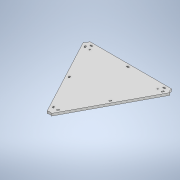
# Autodesk Inventor part: bcc_face
Saved by Autodesk Inventor 2020 (Build 240168000, 168)
## iProperties
Created: 2019-09-26
Part Number: bcc_face
Material: Generic
Document SubType Name: Modeling
Designer: fabrizio
Density: 1 g/cm^3
Appearance: Default
Author: fabrizio
Autodesk Inventor part; units mm, degrees
ref_plane "YZ Plane" through (0, 0, 0) normal (1, 0, 0) x (0, 1, 0)
ref_plane "XZ Plane" through (0, 0, 0) normal (0, 1, 0) x (-1, 0, 0)
ref_plane "XY Plane" through (0, 0, 0) normal (0, 0, 1) x (1, 0, 0)
sketch "Sketch1" plane through (0, 0, 0) normal (0, 1, 0) x (-1, 0, 0)
  arc A0 (8, 0) -> (3.7667, 7.0578) centre (0, 0) ccw
  arc A1 (154.3333, 7.0578) -> (150.1, 0) centre (158.1, 0) ccw
  arc A2 (75.2833, 141.0622) -> (82.8167, 141.0622) centre (79.05, 148.12) ccw
  circle A3 centre (20.0978, 12.0549) radius 1
  circle A4 centre (138.0022, 12.0549) radius 1
  line L0 (3.7667, 7.0578) -> (75.2833, 141.0622)
  line L1 (82.8167, 141.0622) -> (154.3333, 7.0578)
  line L2 (150.1, 0) -> (8, 0)
  line L3 (14.06, 4) -> (17.56, 4)
  line L4 (17.56, 4) -> (17.56, 6)
  line L5 (17.56, 6) -> (14.06, 6)
  line L6 (14.06, 6) -> (14.06, 4)
  line L7 (77.3, 4) -> (80.8, 4)
  line L8 (80.8, 4) -> (80.8, 6)
  line L9 (80.8, 6) -> (77.3, 6)
  line L10 (77.3, 6) -> (77.3, 4)
  line L11 (140.54, 4) -> (144.04, 4)
  line L12 (144.04, 4) -> (144.04, 6)
  line L13 (144.04, 6) -> (140.54, 6)
  line L14 (140.54, 6) -> (140.54, 4)
  line L15 (11.756, 9.663) -> (13.4039, 12.7508)
  line L16 (13.4039, 12.7508) -> (11.6395, 13.6924)
  line L17 (11.6395, 13.6924) -> (9.9915, 10.6046)
  line L18 (9.9915, 10.6046) -> (11.756, 9.663)
  line L19 (43.376, 68.911) -> (45.0239, 71.9988)
  line L20 (45.0239, 71.9988) -> (43.2595, 72.9404)
  line L21 (43.2595, 72.9404) -> (41.6115, 69.8526)
  line L22 (41.6115, 69.8526) -> (43.376, 68.911)
  line L23 (74.996, 128.159) -> (76.6439, 131.2468)
  line L24 (76.6439, 131.2468) -> (74.8795, 132.1884)
  line L25 (74.8795, 132.1884) -> (73.2315, 129.1006)
  line L26 (73.2315, 129.1006) -> (74.996, 128.159)
  line L27 (144.5388, 12.6668) -> (146.1868, 9.5791)
  line L28 (146.1868, 9.5791) -> (147.9512, 10.5207)
  line L29 (147.9512, 10.5207) -> (146.3033, 13.6085)
  line L30 (146.3033, 13.6085) -> (144.5388, 12.6668)
  line L31 (112.9188, 71.9148) -> (114.5668, 68.8271)
  line L32 (114.5668, 68.8271) -> (116.3312, 69.7687)
  line L33 (116.3312, 69.7687) -> (114.6833, 72.8565)
  line L34 (114.6833, 72.8565) -> (112.9188, 71.9148)
  line L35 (81.2988, 131.1628) -> (82.9468, 128.0751)
  line L36 (82.9468, 128.0751) -> (84.7112, 129.0167)
  line L37 (84.7112, 129.0167) -> (83.0633, 132.1045)
  line L38 (83.0633, 132.1045) -> (81.2988, 131.1628)
  point P0 (150.1, 0)
  point P1 (154.3333, 7.0578)
  constraints: 78 end point, 6 point on circle, 5 centre point
extrude "Extrusion1" add sketch "Sketch1" along normal blind 4
body "Solid1"
